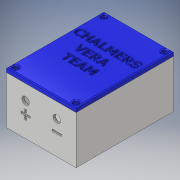
# Autodesk Inventor part: Box
Saved by Autodesk Inventor 2019.3 (Build 233278000, 278)
## iProperties
Created: 2019-02-26
Part Number: Box
Material: Generic
Document SubType Name: Modeling
Designer: oskar
Density: 1 g/cm^3
Appearance: Default
Author: oskar
## iProperties of the stored document Box_3DPrint.ipt
Created: 2019-02-26
Part Number: Box_3DPrint
Material: Generic
Document SubType Name: Modeling
Designer: oskar
Density: 1 g/cm^3
Appearance: Default
Author: oskar
Autodesk Inventor part; units mm, degrees
ref_plane "YZ Plane" through (0, 0, 0) normal (1, 0, 0) x (0, 1, 0)
ref_plane "XZ Plane" through (0, 0, 0) normal (0, 1, 0) x (-1, 0, 0)
ref_plane "XY Plane" through (0, 0, 0) normal (0, 0, 1) x (1, 0, 0)
sketch "Sketch1" plane through (0, 0, 0) normal (0, 1, 0) x (-1, 0, 0)
  line L0 (-35, 50) -> (35, 50)
  line L1 (35, 50) -> (35, -50)
  line L2 (35, -50) -> (-35, -50)
  line L3 (-35, -50) -> (-35, 50)
  line L4 (-35, 50) -> (35, -50) construction
  line L5 (35, 50) -> (-35, -50) construction
  line L6 (-37.4, 52.4) -> (37.4, 52.4)
  line L7 (37.4, 52.4) -> (37.4, -52.4)
  line L8 (37.4, -52.4) -> (-37.4, -52.4)
  line L9 (-37.4, -52.4) -> (-37.4, 52.4)
  line L10 (-37.4, 52.4) -> (37.4, -52.4) construction
  line L11 (37.4, 52.4) -> (-37.4, -52.4) construction
  point P0 (0, 0)
  dimension "d0" = 100
  dimension "d1" = 70
  dimension "d2" = 2.4
  dimension "d3" = 2.4
  constraints: 24 end point, 4 midpoint, 4 parallel, 2 horizontal, 2 perpendicular
  measures "d0" distance of L0.end L1.end
  measures "d1" distance of L1.end L2.end
  measures "d2" distance between parallel lines of L7 L1
  measures "d3" distance between parallel lines of L8 L2
extrude "Extrusion1" add sketch "Sketch1" along normal blind 50
extrude "Extrusion2" add sketch "Sketch1" against normal blind 2.4 contours L0 L1 L2 L3 | L6 L7 L8 L9
sketch "Sketch2" plane through (-37.4, 50, 52.4) normal (0, 0, 1) x (1, 0, 0)
  line L0 (0, 14.8174) -> (0, -75.0826) construction
  line L1 (37.4, 15.8174) -> (37.4, -74.0826) construction
  line L2 (74.8, 14.4373) -> (74.8, -75.4627) construction
  line L3 (74.8, -52.4) -> (74.8, 0) projected
  line L4 (0, 0) -> (0, -52.4) projected
  circle A0 centre (54.2405, -16) radius 4
  circle A1 centre (20.5595, -16) radius 4
  line L5 (0, 0) -> (74.8, 0) projected
  point P0 (37.4, -50)
  dimension "d8" = 8
  dimension "d9" = 16
  constraints: 6 end point, 3 vertical, 2 centre point, 2 collinear, 1 symmetric about line, 2 other
  measures "d8" diameter of A0
  measures "d9" distance from line of L5 A0.centre
extrude "Extrusion3" cut sketch "Sketch2" against normal up to surface (104.8 mm away)
sketch "Sketch3" plane through (-37.4, 50, -52.4) normal (-1, 0, 0) x (0, 0, 1)
  line L0 (104.8, -12) -> (104.8, -20) projected
  line L1 (91.6887, -16) -> (56.9987, -16) construction
  circle A0 centre (53, -16) radius 6
  circle A1 centre (79.9052, -16) radius 3
  circle A2 centre (21.801, -16) radius 3.5
  point P0 (52.4, -50)
  dimension "d12" = 12
  dimension "d15" = 6
  dimension "d16" = 7
  constraints: 3 centre point, 2 end point, 2 point on line, 1 horizontal
  measures "d12" diameter of A0
  measures "d15" diameter of A1
  measures "d16" diameter of A2
extrude "Extrusion4" cut sketch "Sketch3" against normal up to next
sketch "Sketch5" plane through (-35, 50, -50) normal (0, 0, 1) x (1, 0, 0)
  line L0 (30, -31) -> (60, -31)
  line L1 (60, -31) -> (60, -46)
  line L2 (60, -46) -> (30, -46)
  line L3 (30, -46) -> (30, -31)
  line L4 (30, -31) -> (60, -46) construction
  line L5 (60, -31) -> (30, -46) construction
  line L6 (70, -50) -> (70, 0) projected
  line L7 (70, -50) -> (0, -50) projected
  point P0 (35, -50)
  point P1 (45, -38.5)
  dimension "d17" = 10
  dimension "d18" = 4
  dimension "d20" = 15
  dimension "d21" = 30
  constraints: 12 end point, 2 midpoint, 2 parallel, 1 horizontal, 1 perpendicular
  measures "d17" distance between parallel lines of L1 L6
  measures "d18" distance between parallel lines of L2 L7
  measures "d20" distance of L0.end L1.end
  measures "d21" distance of L0.start L0.end
extrude "Extrusion5" cut sketch "Sketch5" against normal up to next
sketch "Sketch6" plane through (-37.4, 50, 52.4) normal (0, 0, 1) x (1, 0, 0)
  line L0 (49.2405, -30) -> (59.2405, -30)
  line L1 (59.2405, -30) -> (59.2405, -28)
  line L2 (59.2405, -28) -> (49.2405, -28)
  line L3 (49.2405, -28) -> (49.2405, -30)
  line L4 (49.2405, -30) -> (59.2405, -28) construction
  line L5 (59.2405, -30) -> (49.2405, -28) construction
  line L6 (14.3617, -29) -> (20.5595, -29) construction
  circle A0 centre (20.5595, -16) radius 4 projected
  line L7 (15.5595, -30) -> (25.5595, -30)
  line L8 (25.5595, -30) -> (25.5595, -28)
  line L9 (25.5595, -28) -> (15.5595, -28)
  line L10 (15.5595, -28) -> (15.5595, -30)
  line L11 (15.5595, -30) -> (25.5595, -28) construction
  line L12 (25.5595, -30) -> (15.5595, -28) construction
  line L13 (19.5595, -34) -> (21.5595, -34)
  line L14 (21.5595, -34) -> (21.5595, -24)
  line L15 (21.5595, -24) -> (19.5595, -24)
  line L16 (19.5595, -24) -> (19.5595, -34)
  line L17 (19.5595, -34) -> (21.5595, -24) construction
  line L18 (21.5595, -34) -> (19.5595, -24) construction
  line L19 (20.5595, -16) -> (20.5595, -21.6445) construction
  line L20 (54.2405, -11.6171) -> (54.2405, -19.4612) construction
  circle A1 centre (54.2405, -16) radius 4 projected
  point P0 (37.4, -50)
  point P1 (54.2405, -29)
  point P2 (54.2405, -29)
  point P3 (20.5595, -29)
  dimension "d24" = 2
  dimension "d25" = 10
  dimension "d26" = 2
  dimension "d27" = 2
  dimension "d28" = 10
  dimension "d29" = 10
  dimension "d32" = 8
  constraints: 42 end point, 7 midpoint, 6 parallel, 4 horizontal, 3 perpendicular, 3 point on line, 2 vertical, 1 line through centre
  measures "d24" distance of L0.end L1.end
  measures "d25" distance of L1.end L2.end
  measures "d26" distance of L14.end L15.end
  measures "d27" distance of L7.end L8.end
  measures "d28" distance of L13.end L14.end
  measures "d29" distance of L7.start L7.end
  measures "d32" distance from line of L15 L19.start
extrude "Extrusion6" cut sketch "Sketch6" against normal blind 1.2 contours L3 L2 L1 L0 | L10 L9 L16 L7 | L16 L9 L14 L7 | L7 L14 L13 L16 | L14 L9 L8 L7 | L16 L15 L14 L9
ref_plane "Work Plane1" through (-37.4, 50, 0) normal (0, 0, 1) x (1, 0, 0)
mirror "Mirror1" about plane through (-37.4, 50, 0) normal (0, 0, 1) of "Extrusion6"
sketch "Sketch7" plane through (-37.4, 50, -52.4) normal (-1, 0, 0) x (0, 0, 1)
  line L0 (1.5214, -14.7444) -> (4.7522, -14.7444) construction
  line L1 (4.7522, -14.7444) -> (4.7522, -17.7924) construction
  line L2 (4.7522, -17.7924) -> (1.5214, -17.7924) construction
  line L3 (1.5214, -17.7924) -> (1.5214, -14.7444) construction
  circle A0 centre (21.801, -16) radius 3.5 projected
  line L4 (21.801, -16) -> (6.3156, -16) construction
  line L5 (27.4526, -14.8292) -> (30.6833, -14.8292) construction
  line L6 (30.6833, -14.8292) -> (30.6833, -17.8772) construction
  line L7 (30.6833, -17.8772) -> (27.4526, -17.8772) construction
  line L8 (27.4526, -17.8772) -> (27.4526, -14.8292) construction
  line L9 (70.875, -28.5614) -> (70.875, -20.5647) construction
  line L10 (70.875, -20.5647) -> (74.1058, -20.5647) construction
  line L11 (74.1058, -20.5647) -> (74.1058, -28.5614) construction
  line L12 (74.1058, -28.5614) -> (70.875, -28.5614) construction
  line L13 (86.2425, -28.8325) -> (86.2425, -20.5647) construction
  line L14 (86.2425, -20.5647) -> (89.4732, -20.5647) construction
  line L15 (89.4732, -20.5647) -> (89.4732, -28.8325) construction
  line L16 (89.4732, -28.8325) -> (86.2425, -28.8325) construction
  line L17 (4.952, -17.9303) -> (4.1908, -17.9303)
  line L18 (4.1908, -17.9303) -> (4.1908, -15.9085)
  line L19 (4.1908, -15.9085) -> (3.6371, -17.2135)
  line L20 (3.6371, -17.2135) -> (3.1131, -17.2135)
  line L21 (3.1131, -17.2135) -> (2.5595, -15.9085)
  line L22 (2.5595, -15.9085) -> (2.5595, -17.9303)
  line L23 (2.5595, -17.9303) -> (1.8378, -17.9303)
  line L24 (1.8378, -17.9303) -> (1.8378, -14.8803)
  line L25 (1.8378, -14.8803) -> (2.7201, -14.8803)
  line L26 (2.7201, -14.8803) -> (3.3974, -16.3855)
  line L27 (3.3974, -16.3855) -> (4.0696, -14.8803)
  line L28 (4.0696, -14.8803) -> (4.952, -14.8803)
  line L29 (4.952, -14.8803) -> (4.952, -17.9303)
  spline S0 degree 2 poles (6.8107, -17.6856) (6.7365, -17.7474) (6.6204, -17.8463) (6.5215, -17.8957) knots 0 0 0 1 2 2 2
  spline S1 degree 2 poles (6.5215, -17.8957) (6.4251, -17.9427) (6.2422, -17.9921) (6.0791, -17.9921) knots 0 0 0 1 2 2 2
  spline S2 degree 2 poles (6.0791, -17.9921) (5.7726, -17.9921) (5.3697, -17.5818) (5.3697, -17.2704) knots 0 0 0 1 2 2 2
  spline S3 degree 2 poles (5.3697, -17.2704) (5.3697, -17.0158) (5.5749, -16.6994) (5.7677, -16.608) knots 0 0 0 1 2 2 2
  spline S4 degree 2 poles (5.7677, -16.608) (5.9629, -16.5141) (6.5042, -16.4399) (6.8156, -16.4201) knots 0 0 0 1 2 2 2
  line L30 (6.8156, -16.4201) -> (6.8156, -16.4078)
  spline S5 degree 2 poles (6.8156, -16.4078) (6.8156, -16.2175) (6.5339, -16.0716) (6.2521, -16.0716) knots 0 0 0 1 2 2 2
  spline S6 degree 2 poles (6.2521, -16.0716) (6.126, -16.0716) (5.785, -16.1631) (5.6243, -16.2348) knots 0 0 0 1 2 2 2
  line L31 (5.6243, -16.2348) -> (5.5625, -16.2348)
  line L32 (5.5625, -16.2348) -> (5.5625, -15.6787)
  spline S7 degree 2 poles (5.5625, -15.6787) (5.6688, -15.649) (6.1434, -15.565) (6.3856, -15.565) knots 0 0 0 1 2 2 2
  spline S8 degree 2 poles (6.3856, -15.565) (6.9788, -15.565) (7.5225, -15.9604) (7.5225, -16.3658) knots 0 0 0 1 2 2 2
  line L33 (7.5225, -16.3658) -> (7.5225, -17.9303)
  line L34 (7.5225, -17.9303) -> (6.8107, -17.9303)
  line L35 (6.8107, -17.9303) -> (6.8107, -17.6856)
  line L36 (6.8107, -17.3297) -> (6.8107, -16.8527)
  spline S9 degree 2 poles (6.8107, -16.8527) (6.6278, -16.87) (6.4029, -16.8972) (6.2941, -16.9367) knots 0 0 0 1 2 2 2
  spline S10 degree 2 poles (6.2941, -16.9367) (6.1977, -16.9689) (6.0939, -17.1023) (6.0939, -17.2111) knots 0 0 0 1 2 2 2
  spline S11 degree 2 poles (6.0939, -17.2111) (6.0939, -17.3717) (6.2694, -17.4928) (6.4399, -17.4928) knots 0 0 0 1 2 2 2
  spline S12 degree 2 poles (6.4399, -17.4928) (6.5339, -17.4928) (6.7316, -17.4063) (6.8107, -17.3297) knots 0 0 0 1 2 2 2
  line L37 (10.2067, -17.9303) -> (9.485, -17.9303)
  line L38 (9.485, -17.9303) -> (9.485, -16.7909)
  spline S13 degree 2 poles (9.485, -16.7909) (9.485, -16.65) (9.4628, -16.3732) (9.4331, -16.3089) knots 0 0 0 1 2 2 2
  spline S14 degree 2 poles (9.4331, -16.3089) (9.396, -16.2298) (9.2576, -16.1631) (9.139, -16.1631) knots 0 0 0 1 2 2 2
  spline S15 degree 2 poles (9.139, -16.1631) (9.0525, -16.1631) (8.872, -16.2298) (8.7707, -16.3015) knots 0 0 0 1 2 2 2
  line L39 (8.7707, -16.3015) -> (8.7707, -17.9303)
  line L40 (8.7707, -17.9303) -> (8.0539, -17.9303)
  line L41 (8.0539, -17.9303) -> (8.0539, -15.6292)
  line L42 (8.0539, -15.6292) -> (8.7707, -15.6292)
  line L43 (8.7707, -15.6292) -> (8.7707, -15.8838)
  spline S16 degree 2 poles (8.7707, -15.8838) (8.9462, -15.7355) (9.2799, -15.5674) (9.4825, -15.5674) knots 0 0 0 1 2 2 2
  spline S17 degree 2 poles (9.4825, -15.5674) (9.8335, -15.5674) (10.2067, -16.0123) (10.2067, -16.4325) knots 0 0 0 1 2 2 2
  line L44 (10.2067, -16.4325) -> (10.2067, -17.9303)
  line L45 (12.8736, -17.9303) -> (12.1568, -17.9303)
  line L46 (12.1568, -17.9303) -> (12.1568, -17.6757)
  spline S18 degree 2 poles (12.1568, -17.6757) (11.9715, -17.8315) (11.66, -17.9946) (11.445, -17.9946) knots 0 0 0 1 2 2 2
  spline S19 degree 2 poles (11.445, -17.9946) (11.1039, -17.9946) (10.7208, -17.562) (10.7208, -17.127) knots 0 0 0 1 2 2 2
  line L47 (10.7208, -17.127) -> (10.7208, -15.6292)
  line L48 (10.7208, -15.6292) -> (11.4425, -15.6292)
  line L49 (11.4425, -15.6292) -> (11.4425, -16.7711)
  spline S20 degree 2 poles (11.4425, -16.7711) (11.4425, -16.9491) (11.4598, -17.1765) (11.4944, -17.2531) knots 0 0 0 1 2 2 2
  spline S21 degree 2 poles (11.4944, -17.2531) (11.529, -17.3248) (11.665, -17.3989) (11.7886, -17.3989) knots 0 0 0 1 2 2 2
  spline S22 degree 2 poles (11.7886, -17.3989) (11.8627, -17.3989) (12.0703, -17.3248) (12.1568, -17.2605) knots 0 0 0 1 2 2 2
  line L50 (12.1568, -17.2605) -> (12.1568, -15.6292)
  line L51 (12.1568, -15.6292) -> (12.8736, -15.6292)
  line L52 (12.8736, -15.6292) -> (12.8736, -17.9303)
  spline S23 degree 2 poles (14.6903, -17.6856) (14.6161, -17.7474) (14.5, -17.8463) (14.4011, -17.8957) knots 0 0 0 1 2 2 2
  spline S24 degree 2 poles (14.4011, -17.8957) (14.3047, -17.9427) (14.1218, -17.9921) (13.9587, -17.9921) knots 0 0 0 1 2 2 2
  spline S25 degree 2 poles (13.9587, -17.9921) (13.6522, -17.9921) (13.2493, -17.5818) (13.2493, -17.2704) knots 0 0 0 1 2 2 2
  spline S26 degree 2 poles (13.2493, -17.2704) (13.2493, -17.0158) (13.4545, -16.6994) (13.6472, -16.608) knots 0 0 0 1 2 2 2
  spline S27 degree 2 poles (13.6472, -16.608) (13.8425, -16.5141) (14.3838, -16.4399) (14.6952, -16.4201) knots 0 0 0 1 2 2 2
  line L53 (14.6952, -16.4201) -> (14.6952, -16.4078)
  spline S28 degree 2 poles (14.6952, -16.4078) (14.6952, -16.2175) (14.4134, -16.0716) (14.1317, -16.0716) knots 0 0 0 1 2 2 2
  spline S29 degree 2 poles (14.1317, -16.0716) (14.0056, -16.0716) (13.6645, -16.1631) (13.5039, -16.2348) knots 0 0 0 1 2 2 2
  line L54 (13.5039, -16.2348) -> (13.4421, -16.2348)
  line L55 (13.4421, -16.2348) -> (13.4421, -15.6787)
  spline S30 degree 2 poles (13.4421, -15.6787) (13.5484, -15.649) (14.0229, -15.565) (14.2651, -15.565) knots 0 0 0 1 2 2 2
  spline S31 degree 2 poles (14.2651, -15.565) (14.8583, -15.565) (15.4021, -15.9604) (15.4021, -16.3658) knots 0 0 0 1 2 2 2
  line L56 (15.4021, -16.3658) -> (15.4021, -17.9303)
  line L57 (15.4021, -17.9303) -> (14.6903, -17.9303)
  line L58 (14.6903, -17.9303) -> (14.6903, -17.6856)
  line L59 (14.6903, -17.3297) -> (14.6903, -16.8527)
  spline S32 degree 2 poles (14.6903, -16.8527) (14.5074, -16.87) (14.2825, -16.8972) (14.1737, -16.9367) knots 0 0 0 1 2 2 2
  spline S33 degree 2 poles (14.1737, -16.9367) (14.0773, -16.9689) (13.9735, -17.1023) (13.9735, -17.2111) knots 0 0 0 1 2 2 2
  spline S34 degree 2 poles (13.9735, -17.2111) (13.9735, -17.3717) (14.149, -17.4928) (14.3195, -17.4928) knots 0 0 0 1 2 2 2
  spline S35 degree 2 poles (14.3195, -17.4928) (14.4134, -17.4928) (14.6112, -17.4063) (14.6903, -17.3297) knots 0 0 0 1 2 2 2
  line L60 (16.6503, -17.9303) -> (15.9335, -17.9303)
  line L61 (15.9335, -17.9303) -> (15.9335, -14.7444)
  line L62 (15.9335, -14.7444) -> (16.6503, -14.7444)
  line L63 (16.6503, -14.7444) -> (16.6503, -17.9303)
  line L64 (27.4402, -17.8792) -> (28.4709, -14.8292)
  line L65 (28.4709, -14.8292) -> (29.3063, -14.8292)
  line L66 (29.3063, -14.8292) -> (30.337, -17.8792)
  line L67 (30.337, -17.8792) -> (29.5485, -17.8792)
  line L68 (29.5485, -17.8792) -> (29.3582, -17.2563)
  line L69 (29.3582, -17.2563) -> (28.3992, -17.2563)
  line L70 (28.3992, -17.2563) -> (28.2064, -17.8792)
  line L71 (28.2064, -17.8792) -> (27.4402, -17.8792)
  line L72 (29.1901, -16.7027) -> (28.8787, -15.6942)
  line L73 (28.8787, -15.6942) -> (28.5648, -16.7027)
  line L74 (28.5648, -16.7027) -> (29.1901, -16.7027)
  line L75 (32.7344, -17.8792) -> (32.0177, -17.8792)
  line L76 (32.0177, -17.8792) -> (32.0177, -17.6246)
  spline S36 degree 2 poles (32.0177, -17.6246) (31.8323, -17.7803) (31.5209, -17.9434) (31.3058, -17.9434) knots 0 0 0 1 2 2 2
  spline S37 degree 2 poles (31.3058, -17.9434) (30.9648, -17.9434) (30.5817, -17.5109) (30.5817, -17.0759) knots 0 0 0 1 2 2 2
  line L77 (30.5817, -17.0759) -> (30.5817, -15.5781)
  line L78 (30.5817, -15.5781) -> (31.3034, -15.5781)
  line L79 (31.3034, -15.5781) -> (31.3034, -16.72)
  spline S38 degree 2 poles (31.3034, -16.72) (31.3034, -16.8979) (31.3207, -17.1253) (31.3553, -17.2019) knots 0 0 0 1 2 2 2
  spline S39 degree 2 poles (31.3553, -17.2019) (31.3899, -17.2736) (31.5258, -17.3478) (31.6494, -17.3478) knots 0 0 0 1 2 2 2
  spline S40 degree 2 poles (31.6494, -17.3478) (31.7235, -17.3478) (31.9312, -17.2736) (32.0177, -17.2094) knots 0 0 0 1 2 2 2
  line L80 (32.0177, -17.2094) -> (32.0177, -15.5781)
  line L81 (32.0177, -15.5781) -> (32.7344, -15.5781)
  line L82 (32.7344, -15.5781) -> (32.7344, -17.8792)
  spline S41 degree 2 poles (34.1631, -17.9237) (33.7256, -17.9237) (33.3252, -17.5628) (33.3252, -17.1525) knots 0 0 0 1 2 2 2
  line L83 (33.3252, -17.1525) -> (33.3252, -16.0773)
  line L84 (33.3252, -16.0773) -> (33.0508, -16.0773)
  line L85 (33.0508, -16.0773) -> (33.0508, -15.5781)
  line L86 (33.0508, -15.5781) -> (33.3252, -15.5781)
  line L87 (33.3252, -15.5781) -> (33.3252, -14.9206)
  line L88 (33.3252, -14.9206) -> (34.0419, -14.9206)
  line L89 (34.0419, -14.9206) -> (34.0419, -15.5781)
  line L90 (34.0419, -15.5781) -> (34.734, -15.5781)
  line L91 (34.734, -15.5781) -> (34.734, -16.0773)
  line L92 (34.734, -16.0773) -> (34.0419, -16.0773)
  line L93 (34.0419, -16.0773) -> (34.0419, -16.8955)
  spline S42 degree 2 poles (34.0419, -16.8955) (34.0419, -17.0166) (34.0469, -17.197) (34.0765, -17.2687) knots 0 0 0 1 2 2 2
  spline S43 degree 2 poles (34.0765, -17.2687) (34.1062, -17.3404) (34.252, -17.4244) (34.3904, -17.4244) knots 0 0 0 1 2 2 2
  spline S44 degree 2 poles (34.3904, -17.4244) (34.4498, -17.4244) (34.6351, -17.375) (34.6722, -17.3552) knots 0 0 0 1 2 2 2
  line L94 (34.6722, -17.3552) -> (34.734, -17.3552)
  line L95 (34.734, -17.3552) -> (34.734, -17.8594)
  spline S45 degree 2 poles (34.734, -17.8594) (34.6178, -17.8891) (34.3558, -17.9237) (34.1631, -17.9237) knots 0 0 0 1 2 2 2
  spline S46 degree 2 poles (37.2328, -16.7299) (37.2328, -17.2983) (36.6124, -17.9508) (36.0464, -17.9508) knots 0 0 0 1 2 2 2
  spline S47 degree 2 poles (36.0464, -17.9508) (35.4829, -17.9508) (34.8576, -17.2983) (34.8576, -16.7299) knots 0 0 0 1 2 2 2
  spline S48 degree 2 poles (34.8576, -16.7299) (34.8576, -16.1564) (35.4829, -15.5064) (36.0464, -15.5064) knots 0 0 0 1 2 2 2
  spline S49 degree 2 poles (36.0464, -15.5064) (36.61, -15.5064) (37.2328, -16.1589) (37.2328, -16.7299) knots 0 0 0 1 2 2 2
  spline S50 degree 2 poles (36.4988, -16.7348) (36.4988, -16.5297) (36.432, -16.2553) (36.3727, -16.1737) knots 0 0 0 1 2 2 2
  spline S51 degree 2 poles (36.3727, -16.1737) (36.3084, -16.0872) (36.1478, -16.0205) (36.0464, -16.0205) knots 0 0 0 1 2 2 2
  spline S52 degree 2 poles (36.0464, -16.0205) (35.9476, -16.0205) (35.7919, -16.0798) (35.7276, -16.1639) knots 0 0 0 1 2 2 2
  spline S53 degree 2 poles (35.7276, -16.1639) (35.6658, -16.2429) (35.5917, -16.5222) (35.5917, -16.7348) knots 0 0 0 1 2 2 2
  spline S54 degree 2 poles (35.5917, -16.7348) (35.5917, -16.9449) (35.6609, -17.2044) (35.7177, -17.2835) knots 0 0 0 1 2 2 2
  spline S55 degree 2 poles (35.7177, -17.2835) (35.7746, -17.3626) (35.9476, -17.4367) (36.0514, -17.4367) knots 0 0 0 1 2 2 2
  spline S56 degree 2 poles (36.0514, -17.4367) (36.1379, -17.4367) (36.3158, -17.3626) (36.3702, -17.2884) knots 0 0 0 1 2 2 2
  spline S57 degree 2 poles (36.3702, -17.2884) (36.432, -17.2019) (36.4988, -16.9523) (36.4988, -16.7348) knots 0 0 0 1 2 2 2
  spline S58 degree 2 poles (73.3862, -22.1515) (73.3862, -22.5469) (73.2601, -23.1401) (73.1192, -23.3403) knots 0 0 0 1 2 2 2
  spline S59 degree 2 poles (73.1192, -23.3403) (72.9808, -23.5381) (72.5335, -23.7407) (72.2121, -23.7407) knots 0 0 0 1 2 2 2
  spline S60 degree 2 poles (72.2121, -23.7407) (71.8884, -23.7407) (71.4435, -23.5381) (71.3026, -23.3354) knots 0 0 0 1 2 2 2
  spline S61 degree 2 poles (71.3026, -23.3354) (71.1617, -23.1352) (71.0356, -22.5469) (71.0356, -22.1515) knots 0 0 0 1 2 2 2
  spline S62 degree 2 poles (71.0356, -22.1515) (71.0356, -21.7461) (71.1617, -21.1727) (71.3051, -20.9651) knots 0 0 0 1 2 2 2
  spline S63 degree 2 poles (71.3051, -20.9651) (71.4484, -20.7624) (71.9007, -20.5647) (72.2121, -20.5647) knots 0 0 0 1 2 2 2
  spline S64 degree 2 poles (72.2121, -20.5647) (72.5409, -20.5647) (72.9808, -20.7723) (73.1217, -20.9774) knots 0 0 0 1 2 2 2
  spline S65 degree 2 poles (73.1217, -20.9774) (73.2601, -21.1776) (73.3862, -21.7684) (73.3862, -22.1515) knots 0 0 0 1 2 2 2
  spline S66 degree 2 poles (72.6175, -22.1515) (72.6175, -21.5855) (72.4321, -21.1282) (72.2121, -21.1282) knots 0 0 0 1 2 2 2
  spline S67 degree 2 poles (72.2121, -21.1282) (71.9922, -21.1282) (71.8043, -21.5855) (71.8043, -22.1539) knots 0 0 0 1 2 2 2
  spline S68 degree 2 poles (71.8043, -22.1539) (71.8043, -22.7125) (71.9922, -23.1772) (72.2121, -23.1772) knots 0 0 0 1 2 2 2
  spline S69 degree 2 poles (72.2121, -23.1772) (72.4296, -23.1772) (72.6175, -22.7125) (72.6175, -22.1515) knots 0 0 0 1 2 2 2
  line L96 (88.6572, -23.6765) -> (86.6429, -23.6765)
  line L97 (86.6429, -23.6765) -> (86.6429, -23.1451)
  line L98 (86.6429, -23.1451) -> (87.2855, -23.1451)
  line L99 (87.2855, -23.1451) -> (87.2855, -21.5311)
  line L100 (87.2855, -21.5311) -> (86.6429, -21.5311)
  line L101 (86.6429, -21.5311) -> (86.6429, -21.0343)
  spline S70 degree 2 poles (86.6429, -21.0343) (86.7837, -21.0343) (87.063, -20.9972) (87.1471, -20.9577) knots 0 0 0 1 2 2 2
  spline S71 degree 2 poles (87.1471, -20.9577) (87.2435, -20.9082) (87.3522, -20.7426) (87.3621, -20.619) knots 0 0 0 1 2 2 2
  line L102 (87.3621, -20.619) -> (88.0294, -20.619)
  line L103 (88.0294, -20.619) -> (88.0294, -23.1451)
  line L104 (88.0294, -23.1451) -> (88.6572, -23.1451)
  line L105 (88.6572, -23.1451) -> (88.6572, -23.6765)
  spline S72 degree 2 poles (91.4255, -22.1515) (91.4255, -22.5469) (91.2994, -23.1401) (91.1585, -23.3403) knots 0 0 0 1 2 2 2
  spline S73 degree 2 poles (91.1585, -23.3403) (91.0201, -23.5381) (90.5728, -23.7407) (90.2514, -23.7407) knots 0 0 0 1 2 2 2
  spline S74 degree 2 poles (90.2514, -23.7407) (89.9277, -23.7407) (89.4828, -23.5381) (89.3419, -23.3354) knots 0 0 0 1 2 2 2
  spline S75 degree 2 poles (89.3419, -23.3354) (89.201, -23.1352) (89.075, -22.5469) (89.075, -22.1515) knots 0 0 0 1 2 2 2
  spline S76 degree 2 poles (89.075, -22.1515) (89.075, -21.7461) (89.201, -21.1727) (89.3444, -20.9651) knots 0 0 0 1 2 2 2
  spline S77 degree 2 poles (89.3444, -20.9651) (89.4877, -20.7624) (89.94, -20.5647) (90.2514, -20.5647) knots 0 0 0 1 2 2 2
  spline S78 degree 2 poles (90.2514, -20.5647) (90.5802, -20.5647) (91.0201, -20.7723) (91.161, -20.9774) knots 0 0 0 1 2 2 2
  spline S79 degree 2 poles (91.161, -20.9774) (91.2994, -21.1776) (91.4255, -21.7684) (91.4255, -22.1515) knots 0 0 0 1 2 2 2
  spline S80 degree 2 poles (90.6568, -22.1515) (90.6568, -21.5855) (90.4714, -21.1282) (90.2514, -21.1282) knots 0 0 0 1 2 2 2
  spline S81 degree 2 poles (90.2514, -21.1282) (90.0315, -21.1282) (89.8436, -21.5855) (89.8436, -22.1539) knots 0 0 0 1 2 2 2
  spline S82 degree 2 poles (89.8436, -22.1539) (89.8436, -22.7125) (90.0315, -23.1772) (90.2514, -23.1772) knots 0 0 0 1 2 2 2
  spline S83 degree 2 poles (90.2514, -23.1772) (90.469, -23.1772) (90.6568, -22.7125) (90.6568, -22.1515) knots 0 0 0 1 2 2 2
  spline S84 degree 2 poles (94.0973, -22.1515) (94.0973, -22.5469) (93.9713, -23.1401) (93.8304, -23.3403) knots 0 0 0 1 2 2 2
  spline S85 degree 2 poles (93.8304, -23.3403) (93.692, -23.5381) (93.2446, -23.7407) (92.9233, -23.7407) knots 0 0 0 1 2 2 2
  spline S86 degree 2 poles (92.9233, -23.7407) (92.5995, -23.7407) (92.1546, -23.5381) (92.0137, -23.3354) knots 0 0 0 1 2 2 2
  spline S87 degree 2 poles (92.0137, -23.3354) (91.8728, -23.1352) (91.7468, -22.5469) (91.7468, -22.1515) knots 0 0 0 1 2 2 2
  spline S88 degree 2 poles (91.7468, -22.1515) (91.7468, -21.7461) (91.8728, -21.1727) (92.0162, -20.9651) knots 0 0 0 1 2 2 2
  spline S89 degree 2 poles (92.0162, -20.9651) (92.1596, -20.7624) (92.6119, -20.5647) (92.9233, -20.5647) knots 0 0 0 1 2 2 2
  spline S90 degree 2 poles (92.9233, -20.5647) (93.252, -20.5647) (93.692, -20.7723) (93.8329, -20.9774) knots 0 0 0 1 2 2 2
  spline S91 degree 2 poles (93.8329, -20.9774) (93.9713, -21.1776) (94.0973, -21.7684) (94.0973, -22.1515) knots 0 0 0 1 2 2 2
  spline S92 degree 2 poles (93.3286, -22.1515) (93.3286, -21.5855) (93.1433, -21.1282) (92.9233, -21.1282) knots 0 0 0 1 2 2 2
  spline S93 degree 2 poles (92.9233, -21.1282) (92.7033, -21.1282) (92.5155, -21.5855) (92.5155, -22.1539) knots 0 0 0 1 2 2 2
  spline S94 degree 2 poles (92.5155, -22.1539) (92.5155, -22.7125) (92.7033, -23.1772) (92.9233, -23.1772) knots 0 0 0 1 2 2 2
  spline S95 degree 2 poles (92.9233, -23.1772) (93.1408, -23.1772) (93.3286, -22.7125) (93.3286, -22.1515) knots 0 0 0 1 2 2 2
  point P0 (52.4, -50)
  constraints: 2 end point, 1 collinear, 1 horizontal, 8 other
extrude "Extrusion7" cut sketch "Sketch7" against normal blind 1.2 contours L17 L18 L19 L20 L21 L22 L23 L24 L25 L26 L27 L28 L29 | S0 S1 S2 S3 S4 L30 S5 S6 L31 L32 S7 S8 L33 L34 L35 | L37 L38 S13 S14 S15 L39 L40 L41 L42 L43 S16 S17 L44 | L45 L46 S18 S19 L47 L48 L49 S20 S21 S22 L50 L51 L52 | S23 S24 S25 S26 S27 L53 S28 S29 L54 L55 S30 S31 L56 L57 L58 | L60 L61 L62 L63 | L64 L65 L66 L67 L68 L69 L70 L71 | L75 L76 S36 S37 L77 L78 L79 S38 S39 S40 L80 L81 L82 | S41 L83 L84 L85 L86 L87 L88 L89 L90 L91 L92 L93 S42 S43 S44 L94 L95 S45 | S46 S47 S48 S49 | S58 S59 S60 S61 S62 S63 S64 S65 | L96 L97 L98 L99 L100 L101 S70 S71 L102 L103 L104 L105 | S72 S73 S74 S75 S76 S77 S78 S79 | S84 S85 S86 S87 S88 S89 S90 S91
sketch "Sketch8" plane through (-37.4, 50, -52.4) normal (-1, 0, 0) x (0, 0, 1)
  point P0 (52.4, -50)
sketch "Sketch9" plane through (0, 50, 0) normal (0, 1, 0) x (1, 0, 0)
  line L0 (35, -50) -> (30, -50)
  line L1 (30, -50) -> (30, -45)
  line L2 (30, -45) -> (35, -45)
  line L3 (35, -45) -> (35, -50)
  line L4 (35, -50) -> (30, -45) construction
  line L5 (30, -50) -> (35, -45) construction
  line L6 (35, -50) -> (-35, -50) construction
  line L7 (35, 50) -> (35, -50) construction
  line L8 (-58.88, 0) -> (56.48, 0) projected
  line L9 (0, 73.36) -> (0, -73.36) projected
  line L10 (-35, -50) -> (-30, -50)
  line L11 (-30, -50) -> (-30, -45)
  line L12 (-30, -45) -> (-35, -45)
  line L13 (-35, -45) -> (-35, -50)
  line L14 (-35, -50) -> (-30, -45) construction
  line L15 (-30, -50) -> (-35, -45) construction
  line L16 (-35, -50) -> (35, -50) construction
  line L17 (-35, 50) -> (-35, -50) construction
  line L18 (35, 50) -> (30, 50)
  line L19 (30, 50) -> (30, 45)
  line L20 (30, 45) -> (35, 45)
  line L21 (35, 45) -> (35, 50)
  line L22 (35, 50) -> (30, 45) construction
  line L23 (30, 50) -> (35, 45) construction
  line L24 (35, 50) -> (-35, 50) construction
  line L25 (-35, 50) -> (-30, 50)
  line L26 (-30, 50) -> (-30, 45)
  line L27 (-30, 45) -> (-35, 45)
  line L28 (-35, 45) -> (-35, 50)
  line L29 (-35, 50) -> (-30, 45) construction
  line L30 (-30, 50) -> (-35, 45) construction
  line L31 (-35, 50) -> (35, 50) construction
  point P0 (0, 0)
  point P1 (32.5, -47.5)
  point P2 (-32.5, -47.5)
  point P3 (32.5, 47.5)
  point P4 (-32.5, 47.5)
  dimension "d35" = 5
  dimension "d36" = 5
  constraints: 56 end point, 22 symmetric about line, 8 midpoint, 2 collinear, 2 parallel, 1 horizontal, 1 perpendicular
  measures "d35" distance of L1.end L2.end
  measures "d36" distance of L0.end L1.end
extrude "Extrusion8" add sketch "Sketch9" against normal blind 10
chamfer "Chamfer1" distance 5 angle 45 8 edges at (35, 40, 47.5) (32.5, 40, 50) (-32.5, 40, 50) (-35, 40, 47.5) (35, 40, -47.5) (32.5, 40, -50) (-35, 40, -47.5) (-32.5, 40, -50)
sketch "Sketch10" plane through (0, 50, 0) normal (0, 1, 0) x (1, 0, 0)
  line L0 (-37.4, 52.4) -> (37.4, 52.4)
  line L1 (37.4, 52.4) -> (37.4, -52.4)
  line L2 (37.4, -52.4) -> (-37.4, -52.4)
  line L3 (-37.4, -52.4) -> (-37.4, 52.4)
  line L4 (-37.4, 52.4) -> (37.4, -52.4) construction
  line L5 (37.4, 52.4) -> (-37.4, -52.4) construction
  line L6 (37.4, -52.4) -> (37.4, 52.4) projected
  line L7 (-37.4, -52.4) -> (37.4, -52.4) projected
  point P0 (0, 0)
  constraints: 12 end point, 2 collinear, 2 midpoint, 2 parallel, 1 horizontal, 1 perpendicular
extrude "Extrusion9" add sketch "Sketch10" along normal blind 4.8 separate body
sketch "Sketch11" plane through (0, 54.8, 0) normal (0, 1, 0) x (1, 0, 0)
  line L0 (30, -45) -> (35, -45) construction
  line L1 (30, -50) -> (30, -45) construction
  line L2 (30, -50) -> (35, -45) construction
  line L3 (30, -45) -> (33.6054, -48.6054) construction
  line L4 (30, -45) -> (35.0989, -45) construction
  line L5 (0, 73.36) -> (0, -73.36) projected
  line L6 (-52.36, 0) -> (52.36, 0) projected
  point P0 (0, 0)
  point P1 (32.5, -47.5)
  point P2 (-32.5, -47.5)
  point P3 (32.5, 47.5)
  point P4 (-32.5, 47.5)
  dimension "d44" = 45
  constraints: 6 end point, 3 symmetric about line, 1 equal length, 1 horizontal, 1 midpoint, 1 point on line
  measures "d44" angle of L3 L4
hole "Hole1" at (32.5, 54.8, 47.5) at (-32.5, 54.8, 47.5) at (32.5, 54.8, -47.5) at (-32.5, 54.8, -47.5) direction (0, -1, 0) diameter 3 depth 54.8 tip angle 118 counterbore diameter 6 counterbore depth 3 bodies 2 1
chamfer "Chamfer2" distance 1 angle 45 12 edges at (-37.4, -2.4, 0) (0, -2.4, 52.4) (37.4, -2.4, 0) (0, -2.4, -52.4) (37.4, 54.8, 0) (0, 54.8, 52.4) (32.5, 54.8, 44.5) (-32.5, 54.8, -50.5) (32.5, 54.8, -50.5) (0, 54.8, -52.4) (-37.4, 54.8, 0) (-32.5, 54.8, 44.5)
chamfer "Chamfer3" distance 5 angle 45 2 edges at (-5, 19, -51.2) (25, 19, -51.2)
sketch "Sketch12" plane through (0, 54.8, 0) normal (0, 1, 0) x (1, 0, 0)
  line L0 (-10.7882, 24.3426) -> (9.6019, 24.3426) construction
  line L1 (9.6019, 24.3426) -> (9.6019, 11.2034) construction
  line L2 (9.6019, 11.2034) -> (-10.7882, 11.2034) construction
  line L3 (-10.7882, 11.2034) -> (-10.7882, 24.3426) construction
  spline S0 degree 2 poles (-30.1677, 14.9925) (-32.1953, 14.9925) (-34.5729, 17.4431) (-34.5729, 19.6603) knots 0 0 0 1 2 2 2
  spline S1 degree 2 poles (-34.5729, 19.6603) (-34.5729, 21.7972) (-32.188, 24.3426) (-30.1604, 24.3426) knots 0 0 0 1 2 2 2
  spline S2 degree 2 poles (-30.1604, 24.3426) (-29.628, 24.3426) (-28.7674, 24.2186) (-28.3736, 24.1165) knots 0 0 0 1 2 2 2
  spline S3 degree 2 poles (-28.3736, 24.1165) (-28.0672, 24.0217) (-27.3452, 23.7081) (-27.1191, 23.5914) knots 0 0 0 1 2 2 2
  line L4 (-27.1191, 23.5914) -> (-27.1191, 21.4472)
  line L5 (-27.1191, 21.4472) -> (-27.3452, 21.4472)
  spline S4 degree 2 poles (-27.3452, 21.4472) (-27.5129, 21.593) (-28.0089, 22.0015) (-28.3225, 22.1911) knots 0 0 0 1 2 2 2
  spline S5 degree 2 poles (-28.3225, 22.1911) (-28.6361, 22.388) (-29.3873, 22.6579) (-29.803, 22.6579) knots 0 0 0 1 2 2 2
  spline S6 degree 2 poles (-29.803, 22.6579) (-30.2917, 22.6579) (-31.1013, 22.3515) (-31.4732, 21.965) knots 0 0 0 1 2 2 2
  spline S7 degree 2 poles (-31.4732, 21.965) (-31.8087, 21.6222) (-32.239, 20.448) (-32.239, 19.653) knots 0 0 0 1 2 2 2
  spline S8 degree 2 poles (-32.239, 19.653) (-32.239, 18.8143) (-31.7941, 17.6692) (-31.4295, 17.3191) knots 0 0 0 1 2 2 2
  spline S9 degree 2 poles (-31.4295, 17.3191) (-31.0794, 16.9763) (-30.2188, 16.6773) (-29.7885, 16.6773) knots 0 0 0 1 2 2 2
  spline S10 degree 2 poles (-29.7885, 16.6773) (-29.3436, 16.6773) (-28.534, 16.9763) (-28.2569, 17.1587) knots 0 0 0 1 2 2 2
  spline S11 degree 2 poles (-28.2569, 17.1587) (-27.9505, 17.341) (-27.4911, 17.7276) (-27.3233, 17.8807) knots 0 0 0 1 2 2 2
  line L6 (-27.3233, 17.8807) -> (-27.1191, 17.8807)
  line L7 (-27.1191, 17.8807) -> (-27.1191, 15.7656)
  spline S12 degree 2 poles (-27.1191, 15.7656) (-27.3671, 15.6489) (-28.0162, 15.3572) (-28.3663, 15.2551) knots 0 0 0 1 2 2 2
  spline S13 degree 2 poles (-28.3663, 15.2551) (-28.7893, 15.1238) (-29.5259, 14.9925) (-30.1677, 14.9925) knots 0 0 0 1 2 2 2
  line L8 (-18.192, 15.1676) -> (-20.453, 15.1676)
  line L9 (-20.453, 15.1676) -> (-20.453, 19.157)
  line L10 (-20.453, 19.157) -> (-23.5235, 19.157)
  line L11 (-23.5235, 19.157) -> (-23.5235, 15.1676)
  line L12 (-23.5235, 15.1676) -> (-25.7844, 15.1676)
  line L13 (-25.7844, 15.1676) -> (-25.7844, 24.1676)
  line L14 (-25.7844, 24.1676) -> (-23.5235, 24.1676)
  line L15 (-23.5235, 24.1676) -> (-23.5235, 20.871)
  line L16 (-23.5235, 20.871) -> (-20.453, 20.871)
  line L17 (-20.453, 20.871) -> (-20.453, 24.1676)
  line L18 (-20.453, 24.1676) -> (-18.192, 24.1676)
  line L19 (-18.192, 24.1676) -> (-18.192, 15.1676)
  line L20 (-17.2949, 15.1676) -> (-14.2536, 24.1676)
  line L21 (-14.2536, 24.1676) -> (-11.7885, 24.1676)
  line L22 (-11.7885, 24.1676) -> (-8.7471, 15.1676)
  line L23 (-8.7471, 15.1676) -> (-11.0737, 15.1676)
  line L24 (-11.0737, 15.1676) -> (-11.6353, 17.0055)
  line L25 (-11.6353, 17.0055) -> (-14.4651, 17.0055)
  line L26 (-14.4651, 17.0055) -> (-15.034, 15.1676)
  line L27 (-15.034, 15.1676) -> (-17.2949, 15.1676)
  line L28 (-12.1313, 18.6392) -> (-13.0502, 21.6149)
  line L29 (-13.0502, 21.6149) -> (-13.9765, 18.6392)
  line L30 (-13.9765, 18.6392) -> (-12.1313, 18.6392)
  line L31 (-1.8476, 15.1676) -> (-7.8501, 15.1676)
  line L32 (-7.8501, 15.1676) -> (-7.8501, 24.1676)
  line L33 (-7.8501, 24.1676) -> (-5.5891, 24.1676)
  line L34 (-5.5891, 24.1676) -> (-5.5891, 16.8815)
  line L35 (-5.5891, 16.8815) -> (-1.8476, 16.8815)
  line L36 (-1.8476, 16.8815) -> (-1.8476, 15.1676)
  line L37 (8.4214, 15.1676) -> (6.1751, 15.1676)
  line L38 (6.1751, 15.1676) -> (6.1751, 21.1335)
  line L39 (6.1751, 21.1335) -> (4.5414, 17.2827)
  line L40 (4.5414, 17.2827) -> (2.9952, 17.2827)
  line L41 (2.9952, 17.2827) -> (1.3615, 21.1335)
  line L42 (1.3615, 21.1335) -> (1.3615, 15.1676)
  line L43 (1.3615, 15.1676) -> (-0.7682, 15.1676)
  line L44 (-0.7682, 15.1676) -> (-0.7682, 24.1676)
  line L45 (-0.7682, 24.1676) -> (1.8355, 24.1676)
  line L46 (1.8355, 24.1676) -> (3.8339, 19.7259)
  line L47 (3.8339, 19.7259) -> (5.8177, 24.1676)
  line L48 (5.8177, 24.1676) -> (8.4214, 24.1676)
  line L49 (8.4214, 24.1676) -> (8.4214, 15.1676)
  line L50 (10.2885, 15.1676) -> (10.2885, 24.1676)
  line L51 (10.2885, 24.1676) -> (16.3712, 24.1676)
  line L52 (16.3712, 24.1676) -> (16.3712, 22.4536)
  line L53 (16.3712, 22.4536) -> (12.5349, 22.4536)
  line L54 (12.5349, 22.4536) -> (12.5349, 20.871)
  line L55 (12.5349, 20.871) -> (16.0722, 20.871)
  line L56 (16.0722, 20.871) -> (16.0722, 19.157)
  line L57 (16.0722, 19.157) -> (12.5349, 19.157)
  line L58 (12.5349, 19.157) -> (12.5349, 16.8815)
  line L59 (12.5349, 16.8815) -> (16.3712, 16.8815)
  line L60 (16.3712, 16.8815) -> (16.3712, 15.1676)
  line L61 (16.3712, 15.1676) -> (10.2885, 15.1676)
  line L62 (26.2172, 15.1676) -> (23.4676, 15.1676)
  line L63 (23.4676, 15.1676) -> (20.966, 18.4715)
  line L64 (20.966, 18.4715) -> (20.1491, 18.4715)
  line L65 (20.1491, 18.4715) -> (20.1491, 15.1676)
  line L66 (20.1491, 15.1676) -> (17.9028, 15.1676)
  line L67 (17.9028, 15.1676) -> (17.9028, 24.1676)
  line L68 (17.9028, 24.1676) -> (21.5203, 24.1676)
  spline S14 degree 2 poles (21.5203, 24.1676) (22.2715, 24.1676) (23.3801, 23.978) (23.8542, 23.6862) knots 0 0 0 1 2 2 2
  spline S15 degree 2 poles (23.8542, 23.6862) (24.3355, 23.3799) (24.9044, 22.4245) (24.9044, 21.6951) knots 0 0 0 1 2 2 2
  spline S16 degree 2 poles (24.9044, 21.6951) (24.9044, 20.6668) (23.9709, 19.3758) (23.1905, 18.9966) knots 0 0 0 1 2 2 2
  line L69 (23.1905, 18.9966) -> (26.2172, 15.1676)
  spline S17 degree 2 poles (22.5851, 21.4107) (22.5851, 21.7535) (22.3226, 22.2421) (22.0235, 22.3734) knots 0 0 0 1 2 2 2
  spline S18 degree 2 poles (22.0235, 22.3734) (21.812, 22.4609) (21.2942, 22.512) (20.9076, 22.512) knots 0 0 0 1 2 2 2
  line L70 (20.9076, 22.512) -> (20.1491, 22.512)
  line L71 (20.1491, 22.512) -> (20.1491, 20.0906)
  line L72 (20.1491, 20.0906) -> (20.7982, 20.0906)
  spline S19 degree 2 poles (20.7982, 20.0906) (21.265, 20.0906) (21.9287, 20.2073) (22.1548, 20.3896) knots 0 0 0 1 2 2 2
  spline S20 degree 2 poles (22.1548, 20.3896) (22.3736, 20.5647) (22.5851, 21.0314) (22.5851, 21.4107) knots 0 0 0 1 2 2 2
  spline S21 degree 2 poles (29.667, 15.0071) (28.6313, 15.0071) (27.0705, 15.4083) (26.3995, 15.7) knots 0 0 0 1 2 2 2
  line L73 (26.3995, 15.7) -> (26.3995, 17.8442)
  line L74 (26.3995, 17.8442) -> (26.6038, 17.8442)
  spline S22 degree 2 poles (26.6038, 17.8442) (27.282, 17.2681) (28.9085, 16.6481) (29.6743, 16.6481) knots 0 0 0 1 2 2 2
  spline S23 degree 2 poles (29.6743, 16.6481) (29.8712, 16.6481) (30.5057, 16.7357) (30.6953, 16.8232) knots 0 0 0 1 2 2 2
  spline S24 degree 2 poles (30.6953, 16.8232) (30.9287, 16.9253) (31.2569, 17.2972) (31.2569, 17.5963) knots 0 0 0 1 2 2 2
  spline S25 degree 2 poles (31.2569, 17.5963) (31.2569, 17.9391) (30.7245, 18.3621) (30.3598, 18.4569) knots 0 0 0 1 2 2 2
  spline S26 degree 2 poles (30.3598, 18.4569) (29.9004, 18.5809) (28.8574, 18.7924) (28.3979, 18.9528) knots 0 0 0 1 2 2 2
  spline S27 degree 2 poles (28.3979, 18.9528) (27.355, 19.3175) (26.4506, 20.5647) (26.4506, 21.4982) knots 0 0 0 1 2 2 2
  spline S28 degree 2 poles (26.4506, 21.4982) (26.4506, 22.76) (28.5875, 24.328) (30.1921, 24.328) knots 0 0 0 1 2 2 2
  spline S29 degree 2 poles (30.1921, 24.328) (30.9944, 24.328) (32.5843, 23.9998) (33.2115, 23.7227) knots 0 0 0 1 2 2 2
  line L75 (33.2115, 23.7227) -> (33.2115, 21.666)
  line L76 (33.2115, 21.666) -> (33.0146, 21.666)
  spline S30 degree 2 poles (33.0146, 21.666) (32.5114, 22.0963) (31.0673, 22.687) (30.3088, 22.687) knots 0 0 0 1 2 2 2
  spline S31 degree 2 poles (30.3088, 22.687) (30.0098, 22.687) (29.543, 22.5995) (29.2804, 22.4828) knots 0 0 0 1 2 2 2
  spline S32 degree 2 poles (29.2804, 22.4828) (29.0689, 22.388) (28.7626, 22.0087) (28.7626, 21.7754) knots 0 0 0 1 2 2 2
  spline S33 degree 2 poles (28.7626, 21.7754) (28.7626, 21.4253) (29.2512, 21.0241) (29.9514, 20.8637) knots 0 0 0 1 2 2 2
  spline S34 degree 2 poles (29.9514, 20.8637) (30.4036, 20.7616) (31.2423, 20.5647) (31.7237, 20.3969) knots 0 0 0 1 2 2 2
  spline S35 degree 2 poles (31.7237, 20.3969) (32.6572, 20.0541) (33.5689, 18.9164) (33.5689, 17.9828) knots 0 0 0 1 2 2 2
  spline S36 degree 2 poles (33.5689, 17.9828) (33.5689, 16.6408) (31.4611, 15.0071) (29.667, 15.0071) knots 0 0 0 1 2 2 2
  line L77 (-10.6726, 9.3493) -> (-13.765, 0.3493)
  line L78 (-13.765, 0.3493) -> (-16.1207, 0.3493)
  line L79 (-16.1207, 0.3493) -> (-19.2131, 9.3493)
  line L80 (-19.2131, 9.3493) -> (-16.8719, 9.3493)
  line L81 (-16.8719, 9.3493) -> (-14.91, 3.2448)
  line L82 (-14.91, 3.2448) -> (-12.9554, 9.3493)
  line L83 (-12.9554, 9.3493) -> (-10.6726, 9.3493)
  line L84 (-9.8338, 0.3493) -> (-9.8338, 9.3493)
  line L85 (-9.8338, 9.3493) -> (-3.7512, 9.3493)
  line L86 (-3.7512, 9.3493) -> (-3.7512, 7.6354)
  line L87 (-3.7512, 7.6354) -> (-7.5875, 7.6354)
  line L88 (-7.5875, 7.6354) -> (-7.5875, 6.0527)
  line L89 (-7.5875, 6.0527) -> (-4.0502, 6.0527)
  line L90 (-4.0502, 6.0527) -> (-4.0502, 4.3388)
  line L91 (-4.0502, 4.3388) -> (-7.5875, 4.3388)
  line L92 (-7.5875, 4.3388) -> (-7.5875, 2.0633)
  line L93 (-7.5875, 2.0633) -> (-3.7512, 2.0633)
  line L94 (-3.7512, 2.0633) -> (-3.7512, 0.3493)
  line L95 (-3.7512, 0.3493) -> (-9.8338, 0.3493)
  line L96 (6.0948, 0.3493) -> (3.3452, 0.3493)
  line L97 (3.3452, 0.3493) -> (0.8436, 3.6532)
  line L98 (0.8436, 3.6532) -> (0.0268, 3.6532)
  line L99 (0.0268, 3.6532) -> (0.0268, 0.3493)
  line L100 (0.0268, 0.3493) -> (-2.2196, 0.3493)
  line L101 (-2.2196, 0.3493) -> (-2.2196, 9.3493)
  line L102 (-2.2196, 9.3493) -> (1.3979, 9.3493)
  spline S37 degree 2 poles (1.3979, 9.3493) (2.1491, 9.3493) (3.2577, 9.1597) (3.7318, 8.868) knots 0 0 0 1 2 2 2
  spline S38 degree 2 poles (3.7318, 8.868) (4.2132, 8.5616) (4.782, 7.6062) (4.782, 6.8769) knots 0 0 0 1 2 2 2
  spline S39 degree 2 poles (4.782, 6.8769) (4.782, 5.8485) (3.8485, 4.5576) (3.0681, 4.1783) knots 0 0 0 1 2 2 2
  line L103 (3.0681, 4.1783) -> (6.0948, 0.3493)
  spline S40 degree 2 poles (2.4628, 6.5924) (2.4628, 6.9352) (2.2002, 7.4239) (1.9012, 7.5552) knots 0 0 0 1 2 2 2
  spline S41 degree 2 poles (1.9012, 7.5552) (1.6897, 7.6427) (1.1718, 7.6937) (0.7853, 7.6937) knots 0 0 0 1 2 2 2
  line L104 (0.7853, 7.6937) -> (0.0268, 7.6937)
  line L105 (0.0268, 7.6937) -> (0.0268, 5.2723)
  line L106 (0.0268, 5.2723) -> (0.6759, 5.2723)
  spline S42 degree 2 poles (0.6759, 5.2723) (1.1427, 5.2723) (1.8064, 5.389) (2.0324, 5.5714) knots 0 0 0 1 2 2 2
  spline S43 degree 2 poles (2.0324, 5.5714) (2.2512, 5.7464) (2.4628, 6.2132) (2.4628, 6.5924) knots 0 0 0 1 2 2 2
  line L107 (5.7958, 0.3493) -> (8.8371, 9.3493)
  line L108 (8.8371, 9.3493) -> (11.3023, 9.3493)
  line L109 (11.3023, 9.3493) -> (14.3436, 0.3493)
  line L110 (14.3436, 0.3493) -> (12.017, 0.3493)
  line L111 (12.017, 0.3493) -> (11.4555, 2.1872)
  line L112 (11.4555, 2.1872) -> (8.6256, 2.1872)
  line L113 (8.6256, 2.1872) -> (8.0568, 0.3493)
  line L114 (8.0568, 0.3493) -> (5.7958, 0.3493)
  line L115 (10.9595, 3.821) -> (10.0405, 6.7966)
  line L116 (10.0405, 6.7966) -> (9.1143, 3.821)
  line L117 (9.1143, 3.821) -> (10.9595, 3.821)
  line L118 (-15.2929, -14.4689) -> (-15.2929, -7.1829)
  line L119 (-15.2929, -7.1829) -> (-17.955, -7.1829)
  line L120 (-17.955, -7.1829) -> (-17.955, -5.4689)
  line L121 (-17.955, -5.4689) -> (-10.3699, -5.4689)
  line L122 (-10.3699, -5.4689) -> (-10.3699, -7.1829)
  line L123 (-10.3699, -7.1829) -> (-13.032, -7.1829)
  line L124 (-13.032, -7.1829) -> (-13.032, -14.4689)
  line L125 (-13.032, -14.4689) -> (-15.2929, -14.4689)
  line L126 (-9.4436, -14.4689) -> (-9.4436, -5.4689)
  line L127 (-9.4436, -5.4689) -> (-3.361, -5.4689)
  line L128 (-3.361, -5.4689) -> (-3.361, -7.1829)
  line L129 (-3.361, -7.1829) -> (-7.1973, -7.1829)
  line L130 (-7.1973, -7.1829) -> (-7.1973, -8.7655)
  line L131 (-7.1973, -8.7655) -> (-3.66, -8.7655)
  line L132 (-3.66, -8.7655) -> (-3.66, -10.4795)
  line L133 (-3.66, -10.4795) -> (-7.1973, -10.4795)
  line L134 (-7.1973, -10.4795) -> (-7.1973, -12.755)
  line L135 (-7.1973, -12.755) -> (-3.361, -12.755)
  line L136 (-3.361, -12.755) -> (-3.361, -14.4689)
  line L137 (-3.361, -14.4689) -> (-9.4436, -14.4689)
  line L138 (-2.7994, -14.4689) -> (0.2419, -5.4689)
  line L139 (0.2419, -5.4689) -> (2.7071, -5.4689)
  line L140 (2.7071, -5.4689) -> (5.7484, -14.4689)
  line L141 (5.7484, -14.4689) -> (3.4218, -14.4689)
  line L142 (3.4218, -14.4689) -> (2.8602, -12.631)
  line L143 (2.8602, -12.631) -> (0.0304, -12.631)
  line L144 (0.0304, -12.631) -> (-0.5385, -14.4689)
  line L145 (-0.5385, -14.4689) -> (-2.7994, -14.4689)
  line L146 (2.3643, -10.9973) -> (1.4453, -8.0216)
  line L147 (1.4453, -8.0216) -> (0.5191, -10.9973)
  line L148 (0.5191, -10.9973) -> (2.3643, -10.9973)
  line L149 (15.8351, -14.4689) -> (13.5888, -14.4689)
  line L150 (13.5888, -14.4689) -> (13.5888, -8.503)
  line L151 (13.5888, -8.503) -> (11.9551, -12.3539)
  line L152 (11.9551, -12.3539) -> (10.4089, -12.3539)
  line L153 (10.4089, -12.3539) -> (8.7752, -8.503)
  line L154 (8.7752, -8.503) -> (8.7752, -14.4689)
  line L155 (8.7752, -14.4689) -> (6.6455, -14.4689)
  line L156 (6.6455, -14.4689) -> (6.6455, -5.4689)
  line L157 (6.6455, -5.4689) -> (9.2492, -5.4689)
  line L158 (9.2492, -5.4689) -> (11.2476, -9.9106)
  line L159 (11.2476, -9.9106) -> (13.2314, -5.4689)
  line L160 (13.2314, -5.4689) -> (15.8351, -5.4689)
  line L161 (15.8351, -5.4689) -> (15.8351, -14.4689)
  point P0 (0, 0)
  constraints: 2 other
extrude "Extrusion10" cut sketch "Sketch12" against normal blind 2.4 bodies 2
equation "\"d0\" = innerLength"
equation "\"d1\" = innerWidth"
equation "\"d2\" = wallThickness"
equation "\"d3\" = wallThickness"
equation "\"d4\" = height"
equation "\"d6\" = wallThickness"
equation "\"d8\" = bananaDiameter"
equation "\"d9\" = 2 * d8"
equation "\"d10\" = wallThickness"
equation "\"d12\" = signalInDiameter"
equation "\"d15\" = switchDiameter"
equation "\"d16\" = potWidth"
equation "\"d26\" = d24"
equation "\"d27\" = d24"
equation "\"d28\" = d25"
equation "\"d29\" = d25"
equation "\"d32\" = bananaDiameter"
equation "\"d30\" = 0.5 * wallThickness"
equation "\"d33\" = 0.5 * wallThickness"
equation "\"d42\" = 2 * wallThickness"
equation "\"d58\" = wallThickness"
equation "\"innerWidth\" = 70"
equation "\"innerLength\" = 100"
equation "\"potWidth\" = 7"
equation "\"wallThickness\" = 2.4"
equation "\"height\" = 50"
equation "\"signalInDiameter\" = 12"
equation "\"bananaDiameter\" = 8"
equation "\"switchDiameter\" = 6"
body "Solid1"
body "Solid2"
